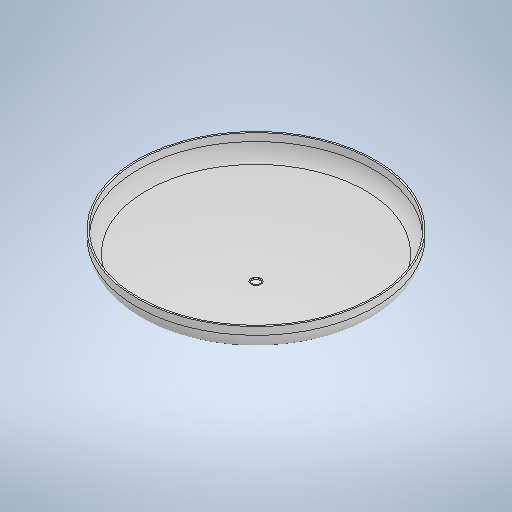
# Autodesk Inventor part: PRS 1604 dished head_D1200 940
Saved by Autodesk Inventor 2026.2 (Build 302298000, 298)
## iProperties
Created: 2025-02-16
Part Number: PRS 1604 dished head_D1200 940
Material: Generic
Document SubType Name: Modeling
Designer: admin
Density: 1 g/cm^3
Appearance: Default
Author: pokla
Autodesk Inventor part; units mm, degrees
ref_plane "YZ Plane" through (0, 0, 0) normal (1, 0, 0) x (0, 1, 0)
ref_plane "XZ Plane" through (0, 0, 0) normal (0, 1, 0) x (-1, 0, 0)
ref_plane "XY Plane" through (0, 0, 0) normal (0, 0, 1) x (1, 0, 0)
sketch "Sketch1" plane through (0, 0, 0) normal (0, 1, 0) x (-1, 0, 0)
  line L0 (470, 0) -> (470, -30)
  arc A0 (432.7406, -89.4136) -> (470, -30) centre (404, -30) ccw
  arc A1 (20, -184) -> (432.7406, -89.4136) centre (20, 763.8182) ccw
  line L1 (0, 0) -> (0, -191.6842)
  arc A2 (20, -178) -> (430.1278, -84.0124) centre (20, 763.8182) ccw
  arc A3 (430.1278, -84.0124) -> (464, -30) centre (404, -30) ccw
  line L2 (464, -30) -> (464, 0)
  line L3 (464, 0) -> (470, 0)
  line L4 (0, -178) -> (0, -184)
  line L5 (0, -184) -> (20, -184)
  line L6 (0, -178) -> (20, -178)
  point P0 (0, 0)
  point P1 (0, -163.7009)
  point P2 (0, -169.7009)
  dimension "d1" = 30
  dimension "d3" = 947.8182
  dimension "d12" = 184
  dimension "d13" = 6
  dimension "d14" = 40
  dimension "d15" = 60
  dimension "d16" = 940
  constraints: 14 end point, 8 point on circle, 4 centre point, 3 horizontal, 3 tangent, 2 vertical, 1 coincident, 1 horizontal alignment, 1 parallel, 1 perpendicular, 1 point on line, 1 vertical alignment, 1 other
  measures "d1" distance of L0.start L0.end
  measures "d3" radius of A1
  measures "d12" distance of L4.end point (0, 0)
  measures "d13" distance of L2.end L0.start
  measures "d14" diameter of L5.end L1
  measures "d15" radius of A3
  measures "d16" diameter of L0 L1
revolve "Revolution1" add sketch "Sketch1" angle 360 about axis through (0, 0, 0) along (0, 0, -1)
sketch "Sketch2" plane through (0, 0, 0) normal (0, 0, 1) x (1, 0, 0)
  circle A0 centre (0, 0) radius 16.75
  dimension "d8" = 33.5
  constraints: 1 centre point, 1 coincident
  measures "d8" diameter of A0
extrude "Extrusion1" cut sketch "Sketch2" against normal through all
equation "\"d12\" = AA_MAIN_dish_hight"
equation "\"d16\" = AA_MAIN_filter_diam"
equation "\"AA_MAIN_filter_diam\" = 940"
equation "\"AA_MAIN_dish_hight\" = 184"
body "Solid1"
